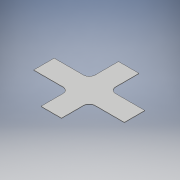
# Autodesk Inventor part: batBox
Saved by Autodesk Inventor 2017 (Build 210142000, 142)
## iProperties
Created: 2017-02-14
Part Number: batBox
Material: Generic
Document SubType Name: Sheet Metal
Designer: kingb
Density: 1 g/cm^3
Sheet Metal Rule: Default
Appearance: Default
Author: kingb
Autodesk Inventor part; units mm, degrees
ref_plane "YZ Plane" through (0, 0, 0) normal (1, 0, 0) x (0, 1, 0)
ref_plane "XZ Plane" through (0, 0, 0) normal (0, 1, 0) x (-1, 0, 0)
ref_plane "XY Plane" through (0, 0, 0) normal (0, 0, 1) x (1, 0, 0)
sketch "Sketch1" plane through (0, 0, 0) normal (0, 1, 0) x (-1, 0, 0)
  line L0 (0, 0) -> (88.9, 0)
  line L1 (88.9, 0) -> (88.9, -95.25)
  line L2 (88.9, -336.55) -> (0, -336.55)
  line L3 (0, -336.55) -> (0, -234.95)
  line L4 (-152.4, -209.55) -> (-25.4, -209.55)
  line L5 (241.3, -209.55) -> (241.3, -120.65)
  line L6 (241.3, -120.65) -> (114.3, -120.65)
  line L7 (-152.4, -120.65) -> (-152.4, -209.55)
  line L8 (88.9, -234.95) -> (88.9, -336.55)
  line L9 (0, -95.25) -> (0, 0)
  line L10 (-25.4, -120.65) -> (-152.4, -120.65)
  line L11 (114.3, -209.55) -> (241.3, -209.55)
  arc A0 (114.3, -209.55) -> (88.9, -234.95) centre (114.3, -234.95) ccw
  arc A1 (0, -234.95) -> (-25.4, -209.55) centre (-25.4, -234.95) ccw
  arc A2 (-25.4, -120.65) -> (0, -95.25) centre (-25.4, -95.25) ccw
  arc A3 (88.9, -95.25) -> (114.3, -120.65) centre (114.3, -95.25) ccw
  point P0 (88.9, -168.275)
  point P1 (88.9, -209.55)
  point P2 (88.9, -120.65)
  point P3 (0, -120.65)
  dimension "d0" = 88.9
  dimension "d1" = 336.55
  dimension "d2" = 393.7
  dimension "d3" = 41.275
  dimension "d4" = 152.4
  dimension "d5" = 88.9
  dimension "d8" = 168.275
  dimension "d9" = 47.625
  dimension "d10" = 120.65
  dimension "d11" = 127
  dimension "d12" = 209.55
  dimension "d13" = 241.3
  dimension "d14" = 25.4
  measures "d0" distance of L2.start L2.end
  measures "d1" distance of L0.end L2.start
  measures "d2" distance of L4.start L5.start
  measures "d3" distance from line of point (88.9, -168.275) L4
  measures "d4" distance from line of L1 L5.start
  measures "d5" distance of L5.start L5.end
  measures "d8" distance from line of L0 point (88.9, -168.275)
  measures "d9" distance of point (88.9, -120.65) point (88.9, -168.275)
  measures "d10" distance of L0.end point (88.9, -120.65)
  measures "d11" distance of point (88.9, -209.55) L2.start
  measures "d12" distance from line of L0 point (88.9, -209.55)
  measures "d13" distance between parallel lines of L5 L9
  measures "d14" radius of A0
extrude "Plate1" add sketch "Sketch1" along normal blind 1.5875
equation "\"BendRadius\" = Thickness"
equation "\"BendReliefWidth\" = Thickness"
equation "\"BendReliefDepth\" = 0.5 * Thickness"
equation "\"CornerReliefSize\" = 4 * Thickness"
equation "\"MinimumRemnant\" = 2 * Thickness"
equation "\"TransitionRadius\" = BendRadius"
equation "\"JacobiRadiusSize\" = Thickness"
equation "\"GapSize\" = Thickness"
equation "\"d15\" = BendRadius"
equation "\"Thickness\" = 1.5875"
body "Solid1"
